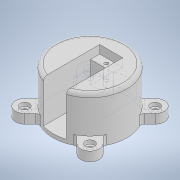
# Autodesk Inventor part: base1
Saved by Autodesk Inventor 2020.2 (Build 242310000, 310)
## iProperties
Created: 2026-05-19
Part Number: base1
Material: Generic
Document SubType Name: Modeling
Designer: explorer
Density: 1 g/cm^3
Appearance: Default
Author: explorer
Autodesk Inventor part; units mm, degrees
ref_plane "YZ Plane" through (0, 0, 0) normal (1, 0, 0) x (0, 1, 0)
ref_plane "XZ Plane" through (0, 0, 0) normal (0, 1, 0) x (-1, 0, 0)
ref_plane "XY Plane" through (0, 0, 0) normal (0, 0, 1) x (1, 0, 0)
sketch "Sketch2" plane through (0, 0, 0) normal (0, 1, 0) x (-1, 0, 0)
  circle A0 centre (0, 0) radius 20
  line L0 (6.25, -6.5) -> (-6.25, -6.5)
  line L1 (-6.25, -6.5) -> (-6.25, 22.6664)
  line L2 (-6.25, 22.6664) -> (6.25, 22.6664)
  line L3 (6.25, 22.6664) -> (6.25, -6.5)
  line L4 (0, -28.5333) -> (0, 31.1997) projected
  line L5 (28, 0) -> (-28, 0) projected
  point P0 (0, -6.5)
  point P1 (6.25, 18.9984)
  point P2 (-6.25, 18.9984)
  dimension "d5" = 40
  dimension "d6" = 6.5
  dimension "d7" = 12.5
  constraints: 8 end point, 2 parallel, 1 centre point, 1 coincident, 1 horizontal, 1 midpoint, 1 perpendicular, 1 point on line
  measures "d5" diameter of A0
  measures "d6" distance from line of L0 point (0, 0)
  measures "d7" distance of L0.start L0.end
extrude "Extrusion1" add sketch "Sketch2" along normal blind 23 contours L5 L3 A0 | A0 L4 L0 L3 L5 | A0 L5 L1 L0 L4 | A0 L1 L5
sketch "Sketch3" plane through (-6.25, 0, -6.5) normal (0, 0, 1) x (1, 0, 0)
  line L0 (0, 23) -> (12.5, 23) projected
  line L1 (0, 23) -> (12.5, 23)
  line L2 (12.5, 23) -> (12.5, 18.5)
  line L3 (12.5, 18.5) -> (0, 18.5)
  line L4 (0, 18.5) -> (0, 23)
  point P0 (0, 0)
  dimension "d10" = 4.5
  constraints: 8 end point, 2 parallel, 1 horizontal, 1 perpendicular
  measures "d10" distance of L0.end L2.end
extrude "Extrusion2" cut sketch "Sketch3" against normal blind 5
sketch "Sketch4" plane through (-6.25, 0, -6.5) normal (0, 0, 1) x (1, 0, 0)
  line L0 (0, 23) -> (12.5, 23)
  line L1 (12.5, 23) -> (12.5, 18.5)
  line L2 (12.5, 18.5) -> (0, 18.5)
  line L3 (0, 18.5) -> (0, 23)
  line L4 (0, 0) -> (10.5075, 0)
  line L5 (0, 0) -> (12.5, 0)
  line L6 (12.5, 0) -> (12.5, 6.5)
  line L7 (12.5, 6.5) -> (0, 6.5)
  line L8 (0, 6.5) -> (0, 0)
  point P0 (6.25, 0)
  point P1 (6.25, 0)
  dimension "d16" = 12
  constraints: 18 end point, 4 coincident, 4 parallel, 2 horizontal, 2 perpendicular
  measures "d16" distance between parallel lines of L7 L2
extrude "Extrusion3" cut sketch "Sketch4" against normal up to surface contours L8 L7 L6 L5 L4 round surface about axis through (0, 0, 0) along (0, 1, 0) radius 20 far side no
sketch "Sketch5" plane through (-6.25, 18.5, -6.5) normal (0, 1, 0) x (1, 0, 0)
  line L0 (12.5, -25.4984) -> (12.5, 12.4984) projected
  line L1 (0, 0) -> (0, 12.4984) projected
  line L2 (0, 0) -> (6.25, 0)
  line L3 (6.25, 0) -> (6.25, 2.4)
  line L4 (6.25, 2.4) -> (0, 2.4)
  line L5 (0, 2.4) -> (0, 0)
  line L6 (12.5, 0) -> (0, 0) projected
  circle A0 centre (6.25, 2.4) radius 1
  point P0 (6.25, -6.5)
  point P1 (12.6412, 0)
  point P2 (12.5, 12.4984)
  dimension "d20" = 2.4
  dimension "d21" = 2
  constraints: 8 end point, 2 parallel, 1 centre point, 1 coincident, 1 horizontal, 1 midpoint, 1 perpendicular, 1 other
  measures "d20" distance from line of L2 L4.end
  measures "d21" diameter of A0
extrude "Extrusion4" cut sketch "Sketch5" against normal blind 8 contours A0 L3 L4 | L4 L3 A0
sketch "Sketch6" plane through (0, 0, 0) normal (0, -1, 0) x (1, 0, 0)
  circle A0 centre (0, 0) radius 20
  constraints: 1 centre point, 1 coincident
extrude "Extrusion5" add sketch "Sketch6" along normal blind 2
sketch "Sketch9" plane through (0, -2, 0) normal (0, -1, 0) x (1, 0, 0)
  line L0 (0, 0) -> (17.6777, 17.6777) construction
  line L1 (0, 0) -> (25, 0) construction
  circle A0 centre (17.6777, 17.6777) radius 1.25
  line L2 (17.6777, 17.6777) -> (21.2132, 14.1421) construction
  arc A1 (21.2132, 14.1421) -> (14.1421, 21.2132) centre (17.6777, 17.6777) ccw
  circle A2 centre (0, 0) radius 20 projected
  line L3 (0, -34.6482) -> (0, 34.6482) projected
  line L4 (-34.6985, 0) -> (34.9497, 0) projected
  line L5 (14.1421, 21.2132) -> (10.1575, 17.2286)
  arc A3 (-6.25, 18.9984) -> (6.25, 18.9984) centre (0, 0) ccw projected
  line L6 (21.2132, 14.1421) -> (17.2286, 10.1575)
  line L7 (-14.1421, 21.2132) -> (-10.1575, 17.2286)
  arc A4 (-14.1421, 21.2132) -> (-21.2132, 14.1421) centre (-17.6777, 17.6777) ccw
  line L8 (-21.2132, 14.1421) -> (-17.2286, 10.1575)
  circle A5 centre (-17.6777, 17.6777) radius 1.25
  line L9 (-21.2132, -14.1421) -> (-17.2286, -10.1575)
  arc A6 (-21.2132, -14.1421) -> (-14.1421, -21.2132) centre (-17.6777, -17.6777) ccw
  line L10 (-14.1421, -21.2132) -> (-10.1575, -17.2286)
  circle A7 centre (-17.6777, -17.6777) radius 1.25
  line L11 (14.1421, -21.2132) -> (10.1575, -17.2286)
  arc A8 (14.1421, -21.2132) -> (21.2132, -14.1421) centre (17.6777, -17.6777) ccw
  line L12 (21.2132, -14.1421) -> (17.2286, -10.1575)
  circle A9 centre (17.6777, -17.6777) radius 1.25
  dimension "d56" = 25
  dimension "d57" = 45
  dimension "d58" = 2.5
  dimension "d59" = 5
  dimension "d62" = 360
  constraints: 22 end point, 10 point on circle, 8 centre point, 5 coincident, 2 parallel, 1 equal length, 1 horizontal, 1 perpendicular, 1 point on line, 41 other
  measures "d56" distance of L0.start L0.end
  measures "d57" angle of L1 L0
  measures "d58" diameter of A0
  measures "d59" distance of L2.start L2.end
extrude "Extrusion8" add sketch "Sketch9" against normal blind 5 contours L6 A2 L5 A1 | L12 A8 L11 A2 | L10 A6 L9 A2 | L8 A4 L7 A2
sketch "Sketch11" plane through (0, 3, 0) normal (0, 1, 0) x (1, 0, 0)
  circle A0 centre (17.6777, -17.6777) radius 1.25 projected
  circle A1 centre (17.6777, -17.6777) radius 2.5
  circle A2 centre (17.6777, 17.6777) radius 2.5
  circle A3 centre (-17.6777, 17.6777) radius 2.5
  circle A4 centre (-17.6777, -17.6777) radius 2.5
  point P0 (0, 0)
  dimension "d66" = 5
  dimension "d69" = 360
  constraints: 4 centre point, 1 coincident, 9 other
  measures "d66" diameter of A1
extrude "Extrusion9" cut sketch "Sketch11" against normal blind 2 contours A0 | A1 | A2 | A3 | A4
fillet "Fillet3" radius 2 1 edges at (0, 23, -20)
fillet "Fillet4" radius 2 10 edges at (-10.1575, 0.5, 17.2286) (10.1575, 1.5, 17.2286) (10.1575, -1, 17.2286) (-17.2286, 0.5, 10.1575) (-17.2286, 0.5, -10.1575) (-10.1575, 0.5, -17.2286) (10.1575, 0.5, -17.2286) (17.2286, 0.5, -10.1575) (17.2286, 1.5, 10.1575) (17.2286, -1, 10.1575)
body "Solid1"
